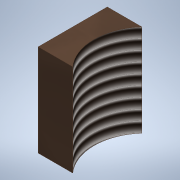
# Autodesk Inventor part: Plaqueta Fosforbronce
Saved by Autodesk Inventor 2020 (Build 240168000, 168)
## iProperties
Created: 2020-09-17
Part Number: Plaqueta Fosforbronce
Material: Bronze
Document SubType Name: Modeling
Designer: aaron
Density: 8.47 g/cm^3
Appearance: Bronze - Satin Hammered
Author: aaron
Autodesk Inventor part; units mm, degrees
ref_plane "YZ Plane" through (0, 0, 0) normal (1, 0, 0) x (0, 1, 0)
ref_plane "XZ Plane" through (0, 0, 0) normal (0, 1, 0) x (-1, 0, 0)
ref_plane "XY Plane" through (0, 0, 0) normal (0, 0, 1) x (1, 0, 0)
sketch "Sketch2" plane through (0, 0, 0) normal (0, 1, 0) x (-1, 0, 0)
  circle A0 centre (0, 0) radius 17.4625
  dimension "d6" = 34.925
  constraints: 2 coincident, 1 centre point
  measures "d6" diameter of A0
extrude "Extrusion2" add sketch "Sketch2" against normal blind 12.7
hole "Hole1" at (0, 0, 0) direction (0, -1, 0) diameter 14.351 end through all thread size "5/8-18 UNF" class "2B" standard "ANSI Unified Screw Threads"
sketch "Sketch3" plane through (0, 0, 0) normal (0, 1, 0) x (1, 0, 0)
  circle A0 centre (0, 0) radius 7.1755 projected
  circle A1 centre (0, 0) radius 7.1755 projected
  circle A2 centre (0, 0) radius 17.4625 projected
  line L0 (-24.4475, 0) -> (24.4475, 0) construction
  line L1 (-5.3672, -4.7625) -> (-10.1297, -4.7625)
  line L2 (-10.1297, -4.7625) -> (-10.1297, 0)
  line L3 (-5.3672, 4.7625) -> (-10.1297, 4.7625)
  line L4 (-10.1297, 4.7625) -> (-10.1297, 0)
  dimension "d16" = 4.7625
  dimension "d17" = 4.7625
  constraints: 8 end point, 2 symmetric about line, 1 horizontal, 1 perpendicular, 1 point on line, 2 other
  measures "d16" distance of L1.end L2.end
  measures "d17" distance of L1.start L1.end
extrude "Extrusion3" cut sketch "Sketch3" against normal blind 12.7 contours A0 L1 L2 L4 L3 keep common part
body "Solid2"
